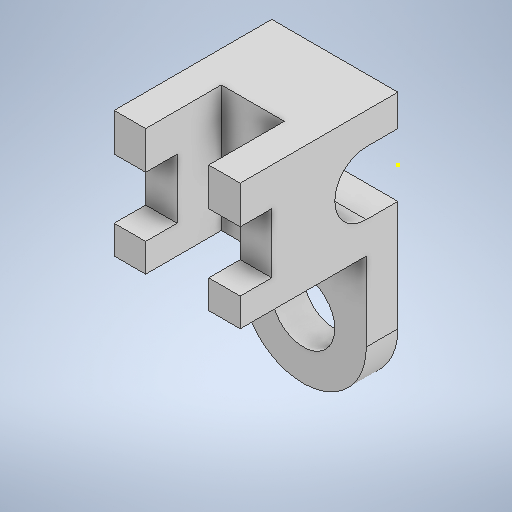
# Autodesk Inventor part: cad@56
Saved by Autodesk Inventor 2025.2 (Build 292293000, 293)
## iProperties
Created: 2025-04-10
Part Number: cad@56
Material: Generic
Document SubType Name: Modeling
Designer: spars
Density: 1 g/cm^3
Appearance: Default
Author: spars
Autodesk Inventor part; units mm, degrees
ref_plane "YZ Plane" through (0, 0, 0) normal (1, 0, 0) x (0, 1, 0)
ref_plane "XZ Plane" through (0, 0, 0) normal (0, 1, 0) x (-1, 0, 0)
ref_plane "XY Plane" through (0, 0, 0) normal (0, 0, 1) x (1, 0, 0)
sketch "Sketch1" plane through (0, 0, 0) normal (0, 0, 1) x (1, 0, 0)
  line L0 (-228.2498, 67.9657) -> (-111.6114, 67.9657) construction
  line L1 (-111.6114, 67.9657) -> (-111.6114, -49.0961) construction
  line L2 (-111.6114, -49.0961) -> (-228.2498, -49.0961) construction
  line L3 (-228.2498, -49.0961) -> (-228.2498, 67.9657) construction
  line L4 (-40, 40) -> (40, 40)
  line L5 (40, 40) -> (40, -40)
  line L6 (40, -40) -> (-40, -40)
  line L7 (-40, -40) -> (-40, 40)
  line L8 (-40, 40) -> (40, -40) construction
  line L9 (40, 40) -> (-40, -40) construction
  point P0 (0, 0)
  dimension "d9" = 80
  dimension "d10" = 80
  constraints: 12 end point, 2 midpoint, 2 parallel, 1 horizontal, 1 perpendicular, 2 other
  measures "d9" distance of L5.end L6.end
  measures "d10" distance of L4.end L5.end
extrude "Extrusion1" add sketch "Sketch1" along normal blind 100
sketch "Sketch2" plane through (40, -40, 0) normal (1, 0, 0) x (0, 0, -1)
  line L0 (-100, 0) -> (-100, 80) projected
  line L1 (-100, 18) -> (-80, 18)
  line L2 (-80, 18) -> (-80, 56)
  line L3 (-80, 56) -> (-100, 56)
  line L4 (-100, 56) -> (-100, 18)
  line L5 (0, 0) -> (-100, 0) projected
  line L6 (0, 80) -> (-100, 80) projected
  point P0 (0, 40)
  dimension "d13" = 20
  dimension "d14" = 38
  dimension "d41" = 24
  constraints: 8 end point, 2 parallel, 1 horizontal, 1 perpendicular, 1 point on line
  measures "d13" distance of L3.end L2.end
  measures "d14" distance of L2.end L1.end
  measures "d41" distance between parallel lines of L6 L3
extrude "Extrusion2" cut sketch "Sketch2" against normal blind 100
sketch "Sketch3" plane through (40, -22, 80) normal (0, 0, 1) x (1, 0, 0)
  point P0 (-40, 22)
sketch "Sketch4" plane through (0, 0, 100) normal (0, 0, 1) x (1, 0, 0)
  line L0 (-40, 40) -> (-40, 16) projected
  point P0 (0, 0)
extrude "Extrusion3" [suppressed]
sketch "Sketch5" plane through (40, -40, 0) normal (1, 0, 0) x (0, 0, -1)
  line L0 (0, 0) -> (0, 80) projected
  line L1 (0, 20) -> (-20, 20)
  line L2 (-20, 60) -> (0, 60)
  line L3 (0, 60) -> (0, 20)
  line L4 (0, 0) -> (-100, 0) projected
  arc A0 (-20, 60) -> (-20, 20) centre (-20, 40) ccw
  point P0 (0, 40)
  point P1 (-10, 20)
  dimension "d22" = 20
  dimension "d23" = 40
  dimension "d24" = 20
  constraints: 6 end point, 2 point on circle, 1 centre point, 1 horizontal, 1 midpoint, 1 parallel, 1 point on line
  measures "d22" distance of L2.start L2.end
  measures "d23" distance of L1.end L2.start
  measures "d24" distance from line of L4 point (-10, 20)
extrude "Extrusion4" cut sketch "Sketch5" against normal through all
sketch "Sketch6" plane through (40, 40, 100) normal (1, 0, 0) x (0, 0, -1)
  point P0 (100, -40)
sketch "Sketch7" plane through (0, 0, 0) normal (0, 0, 1) x (1, 0, 0)
  line L0 (-40, -40) -> (40, -40) projected
  line L1 (-40, -40) -> (40, -40)
  line L2 (40, -40) -> (40, -90)
  line L3 (-40, -90) -> (-40, -40)
  circle A0 centre (0, -90) radius 20
  arc A1 (-40, -90) -> (40, -90) centre (0, -90) ccw
  point P0 (0, 0)
  dimension "d27" = 50
  dimension "d28" = 40
  dimension "d29" = 80
  constraints: 6 end point, 2 centre point, 2 point on circle, 1 coincident, 1 horizontal, 1 parallel, 1 perpendicular
  measures "d27" distance of L1.end L2.end
  measures "d28" diameter of A0
  measures "d29" diameter of A1
extrude "Extrusion5" add sketch "Sketch7" along normal blind 20
sketch "Sketch8" plane through (0, 0, 0) normal (1, 0, 0) x (0, 1, 0)
  line L0 (-40, 20) -> (-40, 100) projected
  line L1 (-90, 20) -> (-40, 20) projected
  line L2 (-57.3614, 29.7732) -> (-44.3145, 46.466)
  point P0 (0, 0)
  constraints: 2 end point
extrude "Rib1" add sketch "Sketch8" along normal mid plane 10 rib yes fills toward (-50.7986, 38.0888) open curves L2
sketch "Sketch9" plane through (0, 0, 100) normal (0, 0, 1) x (1, 0, 0)
  line L0 (40, 40) -> (-40, 40) projected
  line L1 (-40, -40) -> (40, -40) projected
  line L2 (-20, 40) -> (20, 40)
  line L3 (20, 40) -> (20, -40)
  line L4 (20, -40) -> (-20, -40)
  line L5 (-20, -40) -> (-20, 40)
  line L6 (40, 16) -> (40, -22) projected
  point P0 (0, 0)
  point P1 (20, 40)
  dimension "d42" = 40
  dimension "d43" = 20
  constraints: 8 end point, 2 parallel, 2 point on line, 1 horizontal, 1 perpendicular
  measures "d42" distance of L3.end L4.end
  measures "d43" distance between parallel lines of L6 L3
extrude "Extrusion6" cut sketch "Sketch9" against normal blind 48
body "Solid1"
